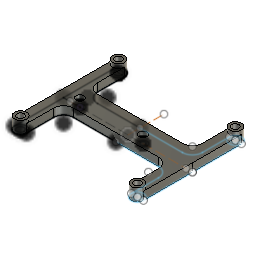
raspi-heatset-mount (Autodesk Fusion 360 design; units mm, degrees)
Autodesk Fusion 360 part; units mm, degrees
sketch "Sketch1" plane through (0, 0, 0) normal (0, 0, 1) x (1, 0, 0)
  circle A0 centre (0, 0) radius 1.2
  circle A1 centre (31.5, 0) radius 1.2
  circle A2 centre (0, 0) radius 2
  circle A3 centre (31.5, 0) radius 2
  circle A4 centre (-5.2276, 24.5) radius 1.725
  line L0 (0, 0) -> (31.5, 0) construction
  line L1 (0, 0) -> (-5, 0) construction
  line L2 (31.5, 0) -> (53, 0) construction
  line L3 (24, 6) -> (2.7724, 6)
  line L4 (-2.2276, 11) -> (-2.2276, 24.5)
  arc A5 (-2.2276, 24.5) -> (-8.2276, 24.5) centre (-5.2276, 24.5) ccw
  line L5 (-5.2276, 24.5) -> (-2.2276, 24.5) construction
  line L6 (-5.2276, 24.5) -> (-8.2276, 24.5) construction
  line L7 (0, 0) -> (-8.2276, 0)
  line L8 (-8.2276, 24.5) -> (-8.2276, 0)
  line L9 (0, 0) -> (-8.2276, 0) construction
  line L10 (24, 0) -> (24, 18) construction
  arc A6 (-2.2276, 11) -> (2.7724, 6) centre (2.7724, 11) ccw
  circle A7 centre (-5.2276, 24.5) radius 3
  line L11 (24, -6) -> (2.7724, -6)
  arc A8 (2.7724, -6) -> (-2.2276, -11) centre (2.7724, -11) ccw
  line L12 (-2.2276, -11) -> (-2.2276, -24.5)
  line L13 (-8.2276, -24.5) -> (-8.2276, 0)
  circle A9 centre (-5.2276, -24.5) radius 3
  circle A10 centre (-5.2276, -24.5) radius 1.725
  line L14 (24, 6) -> (45.2276, 6)
  arc A11 (45.2276, 6) -> (50.2276, 11) centre (45.2276, 11) ccw
  line L15 (50.2276, 11) -> (50.2276, 24.5)
  circle A12 centre (53.2276, 24.5) radius 3
  circle A13 centre (53.2276, 24.5) radius 1.725
  line L16 (56.2276, 24.5) -> (56.2276, 0)
  line L17 (24, -6) -> (45.2276, -6)
  arc A14 (50.2276, -11) -> (45.2276, -6) centre (45.2276, -11) ccw
  line L18 (56.2276, -24.5) -> (56.2276, 0)
  line L19 (50.2276, -11) -> (50.2276, -24.5)
  circle A15 centre (53.2276, -24.5) radius 3
  circle A16 centre (53.2276, -24.5) radius 1.725
  point P0 (24, 0)
  point P1 (-2.2276, 6)
  dimension "d1" = 2.4
  dimension "d2" = 2.4
  dimension "d3" = 31.5
  dimension "d4" = 4
  dimension "d5" = 4
  dimension "d6" = 3.45
  dimension "d15" = 6
  dimension "d22" = 24.5
  dimension "d23" = 3
  dimension "d24" = 3
  dimension "d25" = 26.2276
  dimension "d26" = 5
  dimension "d27" = 8.2276
  constraint coincident A0.centre A2.centre
  constraint concentric A0 A2
  constraint concentric A1 A3
  constraint coincident A1.centre A3.centre
  constraint coincident L2 P0
  constraint perpendicular L3 L4
  constraint coincident A4.centre A5.centre
  constraint perpendicular L4 L5
  constraint perpendicular L6 L8
  constraint perpendicular L8 L9
  constraint coincident P0 L10.start
  constraint perpendicular L0 L10
  constraint coincident P1 L3
  constraint coincident P1 L4
  constraint tangent L3 A6
  constraint tangent L4 A6
  constraint concentric A4 A7
  constraint coincident L4.end A7
  constraint symmetric A4 L0 A10
  constraint symmetric L0 L3.start L11.start
  constraint symmetric L0 L4.end L12.end
  constraint symmetric L0 A5.end L13.start
  constraint symmetric L0 L7.end L8.end
  constraint symmetric L0 L3.end L11.end
  constraint symmetric L0 L4.start A8.end
  constraint symmetric L0 A6 A8
  constraint symmetric L0 A7 A9
  constraint symmetric A4 L10 A13
  constraint symmetric L3.start L10 L14.start
  constraint symmetric L4.end L10 L15.end
  constraint symmetric A5.end L10 L16.start
  constraint symmetric L7.end L10 L16.end
  constraint symmetric L10 L3.end L14.end
  constraint symmetric L10 L4.start A11.end
  constraint symmetric L10 A6 A11
  constraint symmetric L10 A7 A12
  constraint symmetric L10 L11.start L17.start
  constraint symmetric L10 L11.end L17.end
  constraint symmetric L10 A8.end A14.start
  constraint symmetric L10 A8 A14
  constraint symmetric L10 L12.end L19.end
  constraint symmetric L10 L13.start L18.start
  constraint symmetric L10 L7.end L16.end
  constraint symmetric L10 A9 A15
  constraint symmetric L10 A10 A16
  measures "d1" diameter of A0
  measures "d2" diameter of A1
  measures "d3" distance of A0.centre A1.centre
  measures "d4" diameter of A2
  measures "d5" diameter of A3
  measures "d6" diameter of A4
  measures "d15" distance of L0 L3
  measures "d22" distance of A4.centre L7
  measures "d23" distance of A4.centre L4
  measures "d24" horizontal distance of A4.centre A5.end
  measures "d25" distance of L3.start P1
  measures "d26" radius of A6
  measures "d27" distance of A0.centre L8
extrude "Extrude1" add sketch "Sketch1" along normal blind 1 contours A2 | A3 | L3 L4 L8 A6 A7 L11 A8 L12 L13 A9 L14 A11 L15 A12 L16 L17 A14 L18 L19 A15 | A5 A7 | A12 | A9 | A15
extrude "Extrude2" add sketch "Sketch1" along normal blind 4 contours L3 L4 L8 A6 A7 L11 A8 L12 L13 A9 L14 A11 L15 A12 L16 L17 A14 L18 L19 A15
extrude "Extrude3" add sketch "Sketch1" along normal blind 6 contours A5 A7 | A12 | A9 | A15
